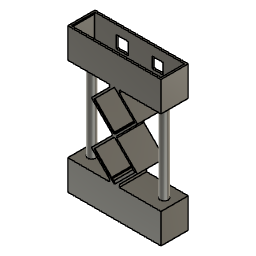
Hourglass Body (Autodesk Fusion 360 design; units mm, degrees)
Autodesk Fusion 360 part; units mm, degrees
note: some values were not read from the file. Set by a fixed rule: which face or edge a step refers to.
sketch "Sketch1" plane through (0, 0, 0) normal (0, 1, 0) x (1, 0, 0)
  line L0 (0, -105.4751) -> (100, -105.4751)
  line L1 (100, -105.4751) -> (100, -75.4751)
  line L2 (0, -75.4751) -> (0, -105.4751)
  line L3 (50, -75.4751) -> (50, -74.4751) construction
  line L4 (50, -74.4751) -> (26.6655, -51.1406)
  line L5 (50, -74.4751) -> (83, -74.4751) construction
  line L6 (26.6655, -51.1406) -> (59.6655, -51.1406) construction
  line L7 (73.3345, -51.1406) -> (50, -74.4751)
  line L8 (73.3345, -51.1406) -> (106.3345, -51.1406) construction
  line L9 (50, -27.806) -> (50, -26.806) construction
  line L10 (50, -26.806) -> (83, -26.806) construction
  line L11 (26.6655, -3.4715) -> (50, 19.863)
  line L12 (50, 19.863) -> (73.3345, -3.4715)
  line L13 (50, 19.863) -> (50, 20.863) construction
  line L14 (100, 20.863) -> (100, 50.863)
  line L15 (100, 50.863) -> (0, 50.863)
  line L16 (0, 50.863) -> (0, 20.863)
  line L17 (0, 20.863) -> (50, 20.863) construction
  line L18 (47.5, 20.863) -> (50, 20.863) construction
  line L19 (47.5, -75.4751) -> (52.5, -75.4751) construction
  line L20 (47.5, -75.4751) -> (50, -75.4751) construction
  line L21 (49, -27.806) -> (51, -27.806) construction
  line L22 (49, -27.806) -> (50, -27.806) construction
  line L23 (49, -27.806) -> (49, -28.806) construction
  line L24 (51, -27.806) -> (51, -28.806) construction
  line L25 (49, -28.806) -> (49, -25.806)
  line L26 (51, -28.806) -> (51, -25.806)
  line L27 (100, -75.4751) -> (52.5, -75.4751)
  line L28 (47.5, -75.4751) -> (0, -75.4751)
  line L29 (0, 20.863) -> (47.5, 20.863)
  line L30 (52.5, 20.863) -> (100, 20.863)
  line L31 (73.3345, -51.1406) -> (51, -28.806)
  line L32 (49, -28.806) -> (26.6655, -51.1406)
  line L33 (73.3345, -3.4715) -> (51, -25.806)
  line L34 (26.6655, -3.4715) -> (49, -25.806)
  line L35 (51, -28.806) -> (49, -28.806)
  line L36 (51, -25.806) -> (49, -25.806)
  line L37 (26.6655, -3.4715) -> (26.6655, 20.863) construction
  line L38 (26.6655, 20.863) -> (0, 20.863) construction
  line L39 (73.3345, -3.4715) -> (73.3345, 20.863) construction
  line L40 (73.3345, 20.863) -> (100, 20.863) construction
  line L41 (50.7929, -29.306) -> (49.2071, -29.306)
  line L42 (49.2071, -29.306) -> (27.3726, -51.1406)
  line L43 (50, -73.768) -> (27.3726, -51.1406)
  line L44 (72.6274, -51.1406) -> (50, -73.768)
  line L45 (72.6274, -51.1406) -> (50.7929, -29.306)
  line L46 (27.3726, -3.4715) -> (49.2071, -25.306)
  line L47 (50.7929, -25.306) -> (49.2071, -25.306)
  line L48 (72.6274, -3.4715) -> (50.7929, -25.306)
  line L49 (50, 19.1559) -> (72.6274, -3.4715)
  line L50 (27.3726, -3.4715) -> (50, 19.1559)
  line L51 (46, -75.4751) -> (54, -75.4751) construction
  line L52 (46, -75.4751) -> (50, -75.4751) construction
  line L53 (46, -75.4751) -> (46, -70.4751)
  line L54 (54, -75.4751) -> (54, -70.4751)
  line L55 (46, 20.863) -> (54, 20.863) construction
  line L56 (46, 20.863) -> (50, 20.863) construction
  line L57 (46, 20.863) -> (46, 15.863)
  line L58 (54, 20.863) -> (54, 15.863)
  dimension "d9" = 100
  dimension "d10" = 30
  dimension "d11" = 1
  dimension "d12" = 135
  dimension "d13" = 33
  dimension "d15" = 33
  dimension "d16" = 33
  dimension "d17" = 135
  dimension "d18" = 33
  dimension "d19" = 1
  dimension "d21" = 33
  dimension "d22" = 33
  dimension "d23" = 33
  dimension "d25" = 1
  dimension "d26" = 100
  dimension "d27" = 30
  dimension "d28" = 5
  dimension "d29" = 5
  dimension "d30" = 2
  dimension "d31" = 47.5
  dimension "d32" = 47.5
  dimension "d33" = 47.5
  dimension "d34" = 47.5
  dimension "d44" = 2
  dimension "d45" = 2
  dimension "d66" = -0.5
  dimension "d67" = 0.5
  dimension "d68" = 8
  dimension "d69" = 8
  constraint horizontal L0
  constraint vertical L1
  constraint vertical L2
  constraint vertical L3
  constraint horizontal L5
  constraint horizontal L6
  constraint horizontal L8
  constraint perpendicular L6 L9
  constraint horizontal L10
  constraint perpendicular L11 L12
  constraint vertical L13
  constraint vertical L14
  constraint horizontal L15
  constraint vertical L16
  constraint perpendicular L3 L19
  constraint midpoint L19 L3.start
  constraint parallel L10 L21
  constraint midpoint L21 L9.start
  constraint perpendicular L21 L23
  constraint perpendicular L21 L24
  constraint parallel L23 L25
  constraint perpendicular L10 L26
  constraint perpendicular L1 L27
  constraint perpendicular L16 L29
  constraint perpendicular L7 L31
  constraint perpendicular L4 L32
  constraint perpendicular L12 L33
  constraint perpendicular L11 L34
  constraint perpendicular L25 L35
  constraint vertical L37
  constraint coincident L29 L37.end
  constraint coincident L17 L37.end
  constraint coincident L30 L39.end
  constraint perpendicular L30 L39
  constraint perpendicular L14 L40
  constraint parallel L19 L51
  constraint midpoint L51 L3.start
  constraint coincident L4 L53.end
  constraint perpendicular L28 L53
  constraint coincident L7 L54.end
  constraint perpendicular L5 L54
  constraint horizontal L55
  constraint midpoint L55 L13.end
  constraint coincident L11 L57.end
  constraint perpendicular L55 L57
  constraint coincident L12 L58.end
  constraint perpendicular L55 L58
  measures "d9" distance of L0.start L0.end
  measures "d10" distance of L0.start L2.start
  measures "d11" distance of L3.start L3.end
  measures "d12" angle of L4 L5
  measures "d13" distance of L3.end L4.end
  measures "d15" distance of L4.end L9.start
  measures "d16" distance of L9.start L7.start
  measures "d17" angle of L7 L8
  measures "d18" distance of L7.start L3.end
  measures "d19" distance of L9.start L9.end
  measures "d21" distance of L9.end L11.start
  measures "d22" distance of L11.start L11.end
  measures "d23" distance of L11.end L12.end
  measures "d25" distance of L11.end L13.end
  measures "d26" distance of L16.end L14.start
  measures "d27" distance of L16.end L15.end
  measures "d28" distance of L18.start L30.start
  measures "d29" distance of L19.start L19.end
  measures "d30" distance of L21.start L21.end
  measures "d31" distance of L1.end L19.end
  measures "d32" distance of L19.start L2.start
  measures "d33" distance of L16.end L18.start
  measures "d34" distance of L30.start L14.start
  measures "d44" distance of L24.end L23.end
  measures "d45" distance of L25.end L26.end
  measures "d68" distance of L51.start L51.end
  measures "d69" distance of L55.start L55.end
extrude "Extrude1" add sketch "Sketch1" along normal blind 30 thin wall 1.5 outside contours L0 L1 L2 L4 L7 L27 L28 L53 L54 | L4 L7 L31 L32 L35 | L25 L26 L35 L36 | L11 L12 L33 L34 L36 | L11 L12 L14 L15 L16 L29 L30 L57 L58 | L41 L42 L43 L44 L45 | L46 L47 L48 L49 L50
extrude "Extrude2" add sketch "Sketch1" along normal blind 1.5 contours L0 L1 L2 L4 L7 L27 L28 L53 L54 | L11 L12 L14 L15 L16 L29 L30 L57 L58
extrude "Extrude3" add sketch "Sketch1" along normal blind 1 contours L25 L26 L35 L36
extrude "Extrude4" add sketch "Sketch1" along normal blind 1 contours L4 L7 L31 L32 L35 | L11 L12 L33 L34 L36
sketch "Sketch2" plane through (0, 0, -19.363) normal (0, 0, 1) x (-1, 0, 0)
  line L0 (1.5, 0) -> (-44.5, 0)
  line L1 (-44.5, -30) -> (1.5, -30)
  line L2 (1.5, -30) -> (1.5, 0)
  line L3 (-21.5, 0) -> (1.5, 0) construction
  line L4 (-10, 0) -> (-10, -30) construction
  circle A0 centre (-10, -15) radius 4.5
  line L5 (-44.5, 0) -> (-44.5, -30)
  dimension "d52" = 9
  constraint midpoint L0 L3.start
  constraint coincident L0.start L2.end
  constraint midpoint L3 L4.start
  constraint coincident L1 L4.end
  constraint perpendicular L1 L4
  constraint midpoint L4 A0.centre
  measures "d52" diameter of A0
sketch "Sketch3" plane through (0, 0, -19.363) normal (0, 0, 1) x (-1, 0, 0)
  line L0 (-55.5, 0) -> (-101.5, 0)
  line L1 (-101.5, 0) -> (-101.5, -30)
  line L2 (-101.5, -30) -> (-55.5, -30)
  line L3 (-101.5, 0) -> (-78.5, 0) construction
  line L4 (-90, 0) -> (-90, -30) construction
  circle A0 centre (-90, -15) radius 4.5
  line L5 (-55.5, -30) -> (-55.5, 0)
  dimension "d56" = 9
  constraint coincident L0.end L1.start
  constraint midpoint L0 L3.end
  constraint midpoint L3 L4.start
  constraint coincident L2 L4.end
  constraint perpendicular L2 L4
  constraint midpoint L4 A0.centre
  measures "d56" diameter of A0
extrude "Extrude5" add sketch "Sketch3" sketch "Sketch2" along normal mid plane 120 from surface at 45 contours A0 of sketch 2 contours A0
sketch "Sketch4" plane through (0, 30, 0) normal (0, 1, 0) x (-1, 0, 0)
  line L0 (-54, -15.863) -> (-73.3345, 3.4715)
  line L1 (-73.3345, 3.4715) -> (-51, 25.806)
  line L2 (-51, 25.806) -> (-51, 28.806)
  line L3 (-51, 28.806) -> (-73.3345, 51.1406)
  line L4 (-73.3345, 51.1406) -> (-54, 70.4751)
  line L5 (-54, 75.4751) -> (-100, 75.4751)
  line L6 (-100, 75.4751) -> (-100, 105.4751)
  line L7 (-100, 105.4751) -> (0, 105.4751)
  line L8 (0, 105.4751) -> (0, 75.4751)
  line L9 (0, 75.4751) -> (-46, 75.4751)
  line L10 (-46, 70.4751) -> (-26.6655, 51.1406)
  line L11 (-26.6655, 51.1406) -> (-49, 28.806)
  line L12 (-49, 28.806) -> (-49, 25.806)
  line L13 (-49, 25.806) -> (-26.6655, 3.4715)
  line L14 (-26.6655, 3.4715) -> (-46, -15.863)
  line L15 (-46, -20.863) -> (0, -20.863)
  line L16 (0, -20.863) -> (0, -50.863)
  line L17 (0, -50.863) -> (-100, -50.863)
  line L18 (-100, -50.863) -> (-100, -20.863)
  line L19 (-100, -20.863) -> (-54, -20.863)
  line L20 (-55.5, -19.363) -> (-101.5, -19.363)
  line L21 (-101.5, -19.363) -> (-101.5, -52.363)
  line L22 (-101.5, -52.363) -> (1.5, -52.363)
  line L23 (1.5, -52.363) -> (1.5, -19.363)
  line L24 (1.5, -19.363) -> (-44.5, -19.363)
  line L25 (-44.5, -16.4843) -> (-24.5442, 3.4715)
  line L26 (-24.5442, 3.4715) -> (-47.5, 26.4274)
  line L27 (-47.5, 26.4274) -> (-47.5, 28.1847)
  line L28 (-47.5, 28.1847) -> (-24.5442, 51.1406)
  line L29 (-24.5442, 51.1406) -> (-44.5, 71.0964)
  line L30 (-44.5, 73.9751) -> (1.5, 73.9751)
  line L31 (1.5, 73.9751) -> (1.5, 106.9751)
  line L32 (1.5, 106.9751) -> (-101.5, 106.9751)
  line L33 (-101.5, 106.9751) -> (-101.5, 73.9751)
  line L34 (-101.5, 73.9751) -> (-55.5, 73.9751)
  line L35 (-55.5, 71.0964) -> (-75.4558, 51.1406)
  line L36 (-75.4558, 51.1406) -> (-52.5, 28.1847)
  line L37 (-52.5, 28.1847) -> (-52.5, 26.4274)
  line L38 (-52.5, 26.4274) -> (-75.4558, 3.4715)
  line L39 (-75.4558, 3.4715) -> (-55.5, -16.4843)
  line L40 (-101.5, -19.363) -> (1.5, -19.363)
  line L41 (1.5, -19.363) -> (1.5, -52.363)
  line L42 (1.5, -52.363) -> (-101.5, -52.363)
  line L43 (-101.5, -52.363) -> (-101.5, -19.363)
  line L44 (-101.5, 106.9751) -> (1.5, 106.9751)
  line L45 (1.5, 106.9751) -> (1.5, 73.9751)
  line L46 (1.5, 73.9751) -> (-101.5, 73.9751)
  line L47 (-101.5, 73.9751) -> (-101.5, 106.9751)
  line L48 (-54, 70.4751) -> (-54, 75.4751)
  line L49 (-46, 75.4751) -> (-46, 70.4751)
  line L50 (-46, -15.863) -> (-46, -20.863)
  line L51 (-54, -20.863) -> (-54, -15.863)
  line L52 (-55.5, -16.4843) -> (-55.5, -19.363)
  line L53 (-44.5, -19.363) -> (-44.5, -16.4843)
  line L54 (-44.5, 71.0964) -> (-44.5, 73.9751)
  line L55 (-55.5, 73.9751) -> (-55.5, 71.0964)
  constraint horizontal L40
  constraint vertical L41
  constraint horizontal L42
  constraint vertical L43
  constraint coincident L22.end L23.start
  constraint coincident L20.end L21.start
  constraint horizontal L44
  constraint vertical L45
  constraint horizontal L46
  constraint vertical L47
  constraint coincident L30.end L31.start
  constraint coincident L32.end L33.start
extrude "Extrude6" add sketch "Sketch4" against normal blind 2 contours L15 L16 L17 L18 L19 L40 L50 L51 | L5 L6 L7 L8 L9 L46 L48 L49
sketch "Sketch5" plane through (0, 0, 106.9751) normal (0, 0, 1) x (-1, 0, 0)
  line L0 (1.5, 0) -> (-101.5, 0)
  line L1 (-101.5, 0) -> (-101.5, -30)
  line L2 (-101.5, -30) -> (1.5, -30)
  line L3 (1.5, -30) -> (1.5, 0)
  line L4 (-99.5, -28) -> (-0.5, -28)
  line L5 (-0.5, -28) -> (-0.5, -2)
  line L6 (-0.5, -2) -> (-99.5, -2)
  line L7 (-99.5, -2) -> (-99.5, -28)
  dimension "d60" = -2
sketch "Sketch6" plane through (0, 0, -52.363) normal (0, 0, -1) x (1, 0, 0)
  line L0 (101.5, 0) -> (-1.5, 0)
  line L1 (-1.5, 0) -> (-1.5, -30)
  line L2 (-1.5, -30) -> (101.5, -30)
  line L3 (101.5, -30) -> (101.5, 0)
  line L4 (99.5, -2) -> (0.5, -2)
  line L5 (0.5, -2) -> (0.5, -28)
  line L6 (0.5, -28) -> (99.5, -28)
  line L7 (99.5, -28) -> (99.5, -2)
  dimension "d61" = -2
extrude "Extrude7" cut sketch "Sketch6" against normal blind 5 contours L4 L5 L6 L7
extrude "Extrude8" cut sketch "Sketch5" against normal blind 5 contours L4 L5 L6 L7
fillet "Fillet1" radius 1.5 12 edges at (54, 15.75, -15.863) (46, 15.75, -15.863) (46, 14.75, -20.863) (54, 14.75, -20.863) (51, 15.5, 25.806) (51, 15.5, 28.806) (49, 15.5, 28.806) (49, 15.5, 25.806) (46, 15.75, 70.4751) (54, 15.75, 70.4751) (54, 14.75, 75.4751) (46, 14.75, 75.4751)
sketch "Sketch7" plane through (0, 30, 0) normal (0, 1, 0) x (-1, 0, 0)
  arc A0 (-54.4393, 70.0358) -> (-54, 71.0964) centre (-55.5, 71.0964) ccw
  line L0 (-54, 71.0964) -> (-54, 73.9751)
  line L1 (-54, 73.9751) -> (-46, 73.9751)
  line L2 (-46, 73.9751) -> (-46, 71.0964)
  arc A1 (-46, 71.0964) -> (-45.5607, 70.0358) centre (-44.5, 71.0964) ccw
  line L3 (-45.5607, 70.0358) -> (-26.6655, 51.1406)
  line L4 (-26.6655, 51.1406) -> (-48.5607, 29.2454)
  arc A2 (-48.5607, 29.2454) -> (-49, 28.1847) centre (-47.5, 28.1847) ccw
  line L5 (-49, 28.1847) -> (-49, 26.4274)
  arc A3 (-49, 26.4274) -> (-48.5607, 25.3667) centre (-47.5, 26.4274) ccw
  line L6 (-48.5607, 25.3667) -> (-26.6655, 3.4715)
  line L7 (-26.6655, 3.4715) -> (-45.5607, -15.4237)
  arc A4 (-45.5607, -15.4237) -> (-46, -16.4843) centre (-44.5, -16.4843) ccw
  line L8 (-46, -16.4843) -> (-46, -19.363)
  line L9 (-46, -19.363) -> (-54, -19.363)
  line L10 (-54, -19.363) -> (-54, -16.4843)
  arc A5 (-54, -16.4843) -> (-54.4393, -15.4237) centre (-55.5, -16.4843) ccw
  line L11 (-54.4393, -15.4237) -> (-73.3345, 3.4715)
  line L12 (-73.3345, 3.4715) -> (-51.4393, 25.3667)
  arc A6 (-51.4393, 25.3667) -> (-51, 26.4274) centre (-52.5, 26.4274) ccw
  line L13 (-51, 26.4274) -> (-51, 28.1847)
  arc A7 (-51, 28.1847) -> (-51.4393, 29.2454) centre (-52.5, 28.1847) ccw
  line L14 (-51.4393, 29.2454) -> (-73.3345, 51.1406)
  line L15 (-73.3345, 51.1406) -> (-54.4393, 70.0358)
  line L16 (-75.4558, 51.1406) -> (-52.5, 28.1847)
  line L17 (-52.5, 28.1847) -> (-52.5, 26.4274)
  line L18 (-52.5, 26.4274) -> (-75.4558, 3.4715)
  line L19 (-75.4558, 3.4715) -> (-55.5, -16.4843)
  line L20 (-55.5, -16.4843) -> (-55.5, -19.363)
  line L21 (-55.5, -19.363) -> (-101.5, -19.363)
  line L22 (-101.5, -19.363) -> (-101.5, -52.363)
  line L23 (-101.5, -52.363) -> (1.5, -52.363)
  line L24 (1.5, -52.363) -> (1.5, -19.363)
  line L25 (1.5, -19.363) -> (-44.5, -19.363)
  line L26 (-44.5, -19.363) -> (-44.5, -16.4843)
  line L27 (-44.5, -16.4843) -> (-24.5442, 3.4715)
  line L28 (-24.5442, 3.4715) -> (-47.5, 26.4274)
  line L29 (-47.5, 26.4274) -> (-47.5, 28.1847)
  line L30 (-47.5, 28.1847) -> (-24.5442, 51.1406)
  line L31 (-24.5442, 51.1406) -> (-44.5, 71.0964)
  line L32 (-44.5, 71.0964) -> (-44.5, 73.9751)
  line L33 (-44.5, 73.9751) -> (1.5, 73.9751)
  line L34 (1.5, 73.9751) -> (1.5, 106.9751)
  line L35 (1.5, 106.9751) -> (-101.5, 106.9751)
  line L36 (-101.5, 106.9751) -> (-101.5, 73.9751)
  line L37 (-101.5, 73.9751) -> (-55.5, 73.9751)
  line L38 (-55.5, 73.9751) -> (-55.5, 71.0964)
  line L39 (-55.5, 71.0964) -> (-75.4558, 51.1406)
  line L40 (-75.75, 96.4751) -> (-63.75, 96.4751)
  line L41 (-63.75, 96.4751) -> (-63.75, 84.4751)
  line L42 (-63.75, 84.4751) -> (-75.75, 84.4751)
  line L43 (-75.75, 84.4751) -> (-75.75, 96.4751)
  line L44 (-75.75, 96.4751) -> (-63.75, 84.4751) construction
  line L45 (-75.75, 84.4751) -> (-63.75, 96.4751) construction
  line L46 (-69.75, 90.4751) -> (-63.75, 90.4751) construction
  line L47 (-37.125, 90.4751) -> (-30.6875, 90.4751) construction
  line L48 (-24.0875, 97.2251) -> (-37.2875, 97.2251)
  line L49 (-37.2875, 97.2251) -> (-37.2875, 83.7251)
  line L50 (-37.2875, 83.7251) -> (-24.0875, 83.7251)
  line L51 (-24.0875, 83.7251) -> (-24.0875, 97.2251)
  line L52 (-24.0875, 97.2251) -> (-37.2875, 83.7251) construction
  line L53 (-37.2875, 97.2251) -> (-24.0875, 83.7251) construction
  line L54 (-101.5, -35.863) -> (1.5, -35.863) construction
  line L55 (-85.5095, -19.363) -> (-85.5095, -52.363) construction
  line L56 (-13.8602, -19.363) -> (-13.8602, -52.363) construction
  line L57 (-89.0095, -29.113) -> (-82.0095, -29.113)
  line L58 (-82.0095, -29.113) -> (-82.0095, -42.613)
  line L59 (-82.0095, -42.613) -> (-89.0095, -42.613)
  line L60 (-89.0095, -42.613) -> (-89.0095, -29.113)
  line L61 (-89.0095, -29.113) -> (-82.0095, -42.613) construction
  line L62 (-82.0095, -29.113) -> (-89.0095, -42.613) construction
  circle A8 centre (-13.8602, -35.863) radius 5.95
  point P0 (-30.6875, 90.4751)
  point P1 (-85.5095, -35.863)
  dimension "d72" = 12
  dimension "d73" = 12
  dimension "d74" = 13.2
  dimension "d75" = 13.5
  dimension "d76" = 7
  dimension "d77" = 13.5
  dimension "d78" = 11.9
  constraint horizontal L40
  constraint vertical L41
  constraint horizontal L42
  constraint vertical L43
  constraint midpoint L45 L46.start
  constraint midpoint L41 L46.end
  constraint horizontal L48
  constraint perpendicular L48 L49
  constraint parallel L48 L50
  constraint parallel L49 L51
  constraint coincident L52 P0
  constraint coincident L53 P0
  constraint coincident P0 L47.end
  constraint midpoint L22 L54.start
  constraint midpoint L24 L54.end
  constraint coincident L21 L55.start
  constraint coincident L23 L55.end
  constraint perpendicular L23 L55
  constraint coincident L25 L56.start
  constraint coincident L23 L56.end
  constraint perpendicular L23 L56
  constraint horizontal L57
  constraint perpendicular L57 L58
  constraint parallel L57 L59
  constraint parallel L58 L60
  constraint coincident L61 P1
  constraint coincident L62 P1
  constraint midpoint L55 P1
  constraint midpoint L56 A8.centre
  measures "d72" distance of L40.start L40.end
  measures "d73" distance of L40.start L42.end
  measures "d74" distance of L49.end L50.end
  measures "d75" distance of L48.end L49.end
  measures "d76" distance of L58.end L59.end
  measures "d77" distance of L57.end L58.end
  measures "d78" diameter of A8
extrude "Extrude9" cut sketch "Sketch7" against normal blind 10 contours L40 L41 L42 L43 | L48 L49 L50 L51 | L57 L58 L59 L60 | A8
sketch "Sketch8" plane through (0, 30, 0) normal (0, 1, 0) x (-1, 0, 0)
  line L0 (-37.2875, 97.2251) -> (-24.0875, 97.2251)
  line L1 (-24.0875, 97.2251) -> (-24.0875, 83.7251)
  line L2 (-24.0875, 83.7251) -> (-37.2875, 83.7251)
  line L3 (-37.2875, 83.7251) -> (-37.2875, 97.2251)
  circle A0 centre (-13.8602, -35.863) radius 5.95
  line L4 (-63.75, 96.4751) -> (-63.75, 84.4751)
  line L5 (-63.75, 84.4751) -> (-75.75, 84.4751)
  line L6 (-75.75, 84.4751) -> (-75.75, 96.4751)
  line L7 (-75.75, 96.4751) -> (-63.75, 96.4751)
  line L8 (-82.0095, -29.113) -> (-82.0095, -42.613)
  line L9 (-82.0095, -42.613) -> (-89.0095, -42.613)
  line L10 (-89.0095, -42.613) -> (-89.0095, -29.113)
  line L11 (-89.0095, -29.113) -> (-82.0095, -29.113)
  arc A1 (-54.4393, 70.0358) -> (-54, 71.0964) centre (-55.5, 71.0964) ccw
  line L12 (-54, 71.0964) -> (-54, 73.9751)
  line L13 (-54, 73.9751) -> (-46, 73.9751)
  line L14 (-46, 73.9751) -> (-46, 71.0964)
  arc A2 (-46, 71.0964) -> (-45.5607, 70.0358) centre (-44.5, 71.0964) ccw
  line L15 (-45.5607, 70.0358) -> (-26.6655, 51.1406)
  line L16 (-26.6655, 51.1406) -> (-48.5607, 29.2454)
  arc A3 (-48.5607, 29.2454) -> (-49, 28.1847) centre (-47.5, 28.1847) ccw
  line L17 (-49, 28.1847) -> (-49, 26.4274)
  arc A4 (-49, 26.4274) -> (-48.5607, 25.3667) centre (-47.5, 26.4274) ccw
  line L18 (-48.5607, 25.3667) -> (-26.6655, 3.4715)
  line L19 (-26.6655, 3.4715) -> (-45.5607, -15.4237)
  arc A5 (-45.5607, -15.4237) -> (-46, -16.4843) centre (-44.5, -16.4843) ccw
  line L20 (-46, -16.4843) -> (-46, -19.363)
  line L21 (-46, -19.363) -> (-54, -19.363)
  line L22 (-54, -19.363) -> (-54, -16.4843)
  arc A6 (-54, -16.4843) -> (-54.4393, -15.4237) centre (-55.5, -16.4843) ccw
  line L23 (-54.4393, -15.4237) -> (-73.3345, 3.4715)
  line L24 (-73.3345, 3.4715) -> (-51.4393, 25.3667)
  arc A7 (-51.4393, 25.3667) -> (-51, 26.4274) centre (-52.5, 26.4274) ccw
  line L25 (-51, 26.4274) -> (-51, 28.1847)
  arc A8 (-51, 28.1847) -> (-51.4393, 29.2454) centre (-52.5, 28.1847) ccw
  line L26 (-51.4393, 29.2454) -> (-73.3345, 51.1406)
  line L27 (-73.3345, 51.1406) -> (-54.4393, 70.0358)
  line L28 (-75.4558, 51.1406) -> (-52.5, 28.1847)
  line L29 (-52.5, 28.1847) -> (-52.5, 26.4274)
  line L30 (-52.5, 26.4274) -> (-75.4558, 3.4715)
  line L31 (-75.4558, 3.4715) -> (-55.5, -16.4843)
  line L32 (-55.5, -16.4843) -> (-55.5, -19.363)
  line L33 (-55.5, -19.363) -> (-101.5, -19.363)
  line L34 (-101.5, -19.363) -> (-101.5, -52.363)
  line L35 (-101.5, -52.363) -> (1.5, -52.363)
  line L36 (1.5, -52.363) -> (1.5, -19.363)
  line L37 (1.5, -19.363) -> (-44.5, -19.363)
  line L38 (-44.5, -19.363) -> (-44.5, -16.4843)
  line L39 (-44.5, -16.4843) -> (-24.5442, 3.4715)
  line L40 (-24.5442, 3.4715) -> (-47.5, 26.4274)
  line L41 (-47.5, 26.4274) -> (-47.5, 28.1847)
  line L42 (-47.5, 28.1847) -> (-24.5442, 51.1406)
  line L43 (-24.5442, 51.1406) -> (-44.5, 71.0964)
  line L44 (-44.5, 71.0964) -> (-44.5, 73.9751)
  line L45 (-44.5, 73.9751) -> (1.5, 73.9751)
  line L46 (1.5, 73.9751) -> (1.5, 106.9751)
  line L47 (1.5, 106.9751) -> (-101.5, 106.9751)
  line L48 (-101.5, 106.9751) -> (-101.5, 73.9751)
  line L49 (-101.5, 73.9751) -> (-55.5, 73.9751)
  line L50 (-55.5, 73.9751) -> (-55.5, 71.0964)
  line L51 (-55.5, 71.0964) -> (-75.4558, 51.1406)
  arc A9 (-46.1, 71.0964) -> (-45.6314, 69.965) centre (-44.5, 71.0964) ccw
  line L52 (-45.6314, 69.965) -> (-26.8069, 51.1406)
  line L53 (-26.8069, 51.1406) -> (-48.6314, 29.3161)
  arc A10 (-48.6314, 29.3161) -> (-49.1, 28.1847) centre (-47.5, 28.1847) ccw
  line L54 (-49.1, 28.1847) -> (-49.1, 26.4274)
  arc A11 (-49.1, 26.4274) -> (-48.6314, 25.296) centre (-47.5, 26.4274) ccw
  line L55 (-48.6314, 25.296) -> (-26.8069, 3.4715)
  line L56 (-26.8069, 3.4715) -> (-45.6314, -15.353)
  arc A12 (-45.6314, -15.353) -> (-46.1, -16.4843) centre (-44.5, -16.4843) ccw
  line L57 (-46.1, -16.4843) -> (-46.1, -19.263)
  line L58 (-46.1, -19.263) -> (-53.9, -19.263)
  line L59 (-53.9, -19.263) -> (-53.9, -16.4843)
  arc A13 (-53.9, -16.4843) -> (-54.3686, -15.353) centre (-55.5, -16.4843) ccw
  line L60 (-54.3686, -15.353) -> (-73.1931, 3.4715)
  line L61 (-73.1931, 3.4715) -> (-51.3686, 25.296)
  arc A14 (-51.3686, 25.296) -> (-50.9, 26.4274) centre (-52.5, 26.4274) ccw
  line L62 (-50.9, 26.4274) -> (-50.9, 28.1847)
  arc A15 (-50.9, 28.1847) -> (-51.3686, 29.3161) centre (-52.5, 28.1847) ccw
  line L63 (-51.3686, 29.3161) -> (-73.1931, 51.1406)
  line L64 (-73.1931, 51.1406) -> (-54.3686, 69.965)
  arc A16 (-54.3686, 69.965) -> (-53.9, 71.0964) centre (-55.5, 71.0964) ccw
  line L65 (-53.9, 71.0964) -> (-53.9, 73.8751)
  line L66 (-53.9, 73.8751) -> (-46.1, 73.8751)
  line L67 (-46.1, 73.8751) -> (-46.1, 71.0964)
  dimension "d81" = 0.1
sketch "Sketch9" plane through (0, 0, 106.9751) normal (0, 0, 1) x (-1, 0, 0)
  line L0 (-0.5, -28) -> (-99.5, -28)
  line L1 (-99.5, -28) -> (-99.5, -2)
  line L2 (-99.5, -2) -> (-0.5, -2)
  line L3 (-0.5, -2) -> (-0.5, -28)
  line L4 (1.5, 0) -> (-101.5, 0)
  line L5 (-101.5, 0) -> (-101.5, -30)
  line L6 (-101.5, -30) -> (1.5, -30)
  line L7 (1.5, -30) -> (1.5, 0)
  line L8 (-99.4, -27.9) -> (-99.4, -2.1)
  line L9 (-99.4, -2.1) -> (-0.6, -2.1)
  line L10 (-0.6, -2.1) -> (-0.6, -27.9)
  line L11 (-0.6, -27.9) -> (-99.4, -27.9)
  dimension "d82" = 0.1
delete_face "DeleteFace1" 4 faces at (5.5224, 15.4481, -25.363) (88.5668, 10.7343, -25.363) (88.7812, 10.6682, 82.2497) (5.5224, 14.5519, 78.8624)
equation "box_length = 10 cm"
equation "box_width = 3 cm"
equation "gap_length_out = 0.5 cm"
equation "gap_width_out = 0.5 cm"
equation "matrix_length = 3.3 cm"
equation "gap_length_in = 0.1 cm"
equation "gap_width_in = 0.2 cm"
equation "thickness = 0.2 cm"
equation "d9 = box_length"
equation "d10 = box_width"
equation "d13 = matrix_length"
equation "d15 = matrix_length"
equation "d16 = matrix_length"
equation "d18 = matrix_length"
equation "d19 = gap_length_in"
equation "d21 = matrix_length"
equation "d22 = matrix_length"
equation "d23 = matrix_length"
equation "d26 = box_length"
equation "d27 = box_width"
equation "d28 = gap_width_out"
equation "d29 = gap_width_out"
equation "d30 = gap_width_in"
equation "d31 = box_length / 2 - gap_length_out / 2"
equation "d32 = box_length / 2 - gap_length_out / 2"
equation "d33 = box_length / 2 - gap_length_out / 2"
equation "d34 = box_length / 2 - gap_length_out / 2"
equation "d44 = gap_width_in"
equation "d45 = gap_width_in"
equation "d52 = hole_diameter"
equation "d56 = hole_diameter"
equation "hole_diameter = 0.9 cm"
